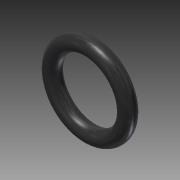
# Autodesk Inventor part: Rubber_Sea_2.5X1N70l##
Saved by Autodesk Inventor 2015 (Build 190159000, 159)
## iProperties
Created: 2015-01-06
Part Number: Rubber_Sea_2.5X1N70l##
Material: Rubber
Document SubType Name: Modeling
Designer: ice
Density: 0.93 g/cm^3
Appearance: Rubber - Black - Version 1.1
Mass: 0.00803139 g
Surface Area: 0.345436 cm^2
Volume: 0.0086359 cm^3
Author: ice
Autodesk Inventor part; units mm, degrees
ref_plane "YZ Plane" through (0, 0, 0) normal (1, 0, 0) x (0, 1, 0)
ref_plane "XZ Plane" through (0, 0, 0) normal (0, 1, 0) x (-1, 0, 0)
ref_plane "XY Plane" through (0, 0, 0) normal (0, 0, 1) x (1, 0, 0)
sketch "Sketch1" plane through (0, 0, 0) normal (0, 0, 1) x (1, 0, 0)
  line L0 (0, -1.5933) -> (0, 3.0491)
  circle A0 centre (2.5, 0) radius 0.5
  point P0 (0, 0)
  dimension "d7" = 1
  dimension "d8" = 2.5
  constraints: 2 end point, 1 centre point, 1 vertical
  measures "d7" diameter of A0
  measures "d8" distance of point (0, 0) A0.centre
revolve "Revolution1" add sketch "Sketch1" angle 360 about axis through (0, -1.5933, 0) along (0, 1, 0)
body "Solid1"
